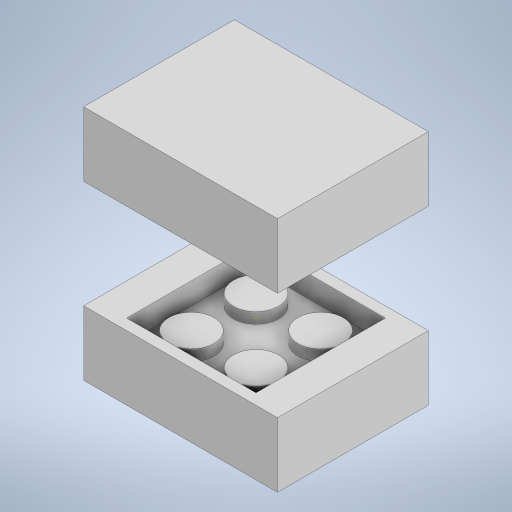
# Autodesk Inventor part: Tercer examen. Cubo LEGO Molde. Villegas
Saved by Autodesk Inventor 2023 (Build 270158000, 158)
## iProperties
Created: 2022-11-04
Part Number: Tercer examen. Cubo LEGO Molde. Villegas
Material: Generic
Document SubType Name: Modeling
Designer: al180794
Density: 1 g/cm^3
Appearance: Default
Author: al180794
Autodesk Inventor part; units mm, degrees
ref_plane "YZ Plane" through (0, 0, 0) normal (1, 0, 0) x (0, 1, 0)
ref_plane "XZ Plane" through (0, 0, 0) normal (0, 1, 0) x (-1, 0, 0)
ref_plane "XY Plane" through (0, 0, 0) normal (0, 0, 1) x (1, 0, 0)
sketch "Sketch2" plane through (0, 0, 0) normal (0, 1, 0) x (-1, 0, 0)
  line L0 (-30, 30) -> (30, 30)
  line L1 (30, 30) -> (30, -30)
  line L2 (30, -30) -> (-30, -30)
  line L3 (-30, -30) -> (-30, 30)
  circle A0 centre (15, 15) radius 10.5
  circle A1 centre (15, -15) radius 10.5
  circle A2 centre (-15, -15) radius 10.5
  circle A3 centre (-15, 15) radius 10.5
  point P0 (0, 0)
  constraints: 8 end point, 4 centre point, 2 parallel, 1 horizontal, 1 perpendicular
extrude "Extrusion1" add sketch "Sketch2" along normal blind 5 and the other way blind 10
extrude "Extrusion2" add sketch "Sketch2" along normal blind 10 and the other way blind 5 contours A0 | A1 | A2 | A3
fillet "Fillet1" radius 0.5 4 edges at (-4.5, 10, 15) (-4.5, 10, -15) (25.5, 10, -15) (25.5, 10, 15)
sketch "Sketch8" plane through (0, 0, 0) normal (0, 0, 1) x (1, 0, 0)
  line L0 (-45, -30) -> (45, -30)
  line L1 (45, -30) -> (45, 30)
  line L2 (45, 30) -> (-45, 30)
  line L3 (-45, -30) -> (45, 30) construction
  line L4 (45, -30) -> (-45, 30) construction
  line L5 (-45, 0.673) -> (-27.6377, 0.673)
  line L6 (-30, 0.673) -> (-30, -2.5)
  line L7 (-30, -2.5) -> (-35.4871, -2.5)
  line L8 (-35.4871, -2.5) -> (-45, -7.327)
  line L9 (-45, -7.327) -> (-45, 0.673)
  line L10 (-45, 30) -> (-45, -30)
  point P0 (0, 0)
  dimension "d39" = 90
  dimension "d40" = 60
  dimension "d41" = 17.3623
  dimension "d42" = 8
  dimension "d43" = 9.5129
  dimension "d44" = 5.4871
  constraints: 22 end point, 2 horizontal, 2 midpoint, 2 perpendicular, 1 parallel, 1 point on line, 1 vertical
  measures "d39" distance of L2.end L1.end
  measures "d40" distance of L1.end L0.end
  measures "d41" distance of L5.start L5.end
  measures "d42" distance of L8.end L5.start
  measures "d43" horizontal distance of L7.end L8.end
  measures "d44" distance of L6.end L7.end
extrude "Extrusion5" add sketch "Sketch8" along normal mid plane 70 separate body
combine bodies "Combine1" operation type subtract main body 2 bodies to subtract 1
split body "Split1" result two bodies by plane through (0, 0, 0) normal (0, 1, 0) bodies 2 first body at (15, 29.5, -11.6667)
move or copy body "Move Body1" bodies to move or copy 3 copy no translate (0, 50, 0)
sketch "Sketch11" plane through (-45, 50, -35) normal (0, -1, 0) x (1, 0, 0)
  line L0 (0, 70) -> (0, 0) projected
  line L1 (0, 30) -> (15, 30)
  line L2 (15, 5) -> (15, 65) projected
  line L3 (15, 38) -> (15, 30)
  line L4 (0, 30) -> (0, 38)
  line L5 (15, 38) -> (0, 38)
  line L6 (15, 38) -> (15, 34)
  line L7 (15, 5) -> (15, 65) projected
  line L8 (15, 34) -> (0, 34)
  line L9 (0, 70) -> (0, 0) projected
  line L10 (0, 0) -> (90, 0) projected
  point P0 (45, 35)
  dimension "d57" = 15
  dimension "d58" = 8
  dimension "d59" = 4
  dimension "d61" = 30
  constraints: 12 end point, 5 point on line, 3 perpendicular, 1 horizontal, 1 vertical
  measures "d57" distance of L3.start L4.end
  measures "d58" distance of L1.start L4.end
  measures "d59" distance of L3.start L6.end
  measures "d61" distance between parallel lines of L10 L1
revolve "Revolution2" cut sketch "Sketch11" angle 180 about axis through (-30, 50, -1) along (1, 0, 0) bodies 3 contours L8 L2 L1 L0
sketch "Sketch12" plane through (-45, 0, -35) normal (0, 1, 0) x (1, 0, 0)
  point P0 (45, -35)
body "Solid3"
body "Solid4"
